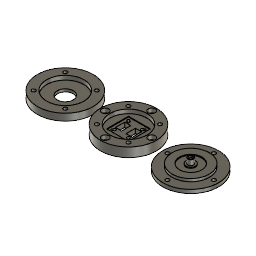
AS5600 holder v2.1 (Autodesk Fusion 360 design; units mm, degrees)
part number: 2026-01-20-22-25-40-409
Autodesk Fusion 360 part; units mm, degrees
sketch "Sketch1" plane through (0, 0, 0) normal (0, 0, 1) x (1, 0, 0)
  circle A0 centre (0, 0) radius 1.9
  circle A1 centre (0, 0) radius 4.9
  circle A2 centre (0, 0) radius 20
  dimension "d1" = 3.8
  dimension "d2" = 9.8
  constraint coincident A0.centre A1.centre
  constraint concentric A0 A1
  constraint concentric A1 A2
  measures "d1" diameter of A0
  measures "d2" diameter of A1
sketch "Sketch2" plane through (0, 0, 0) normal (0, 0, 1) x (1, 0, 0)
  line L0 (30, -30) -> (-30, -30)
  line L1 (-30, -30) -> (-30, 30)
  line L2 (-30, 30) -> (30, 30)
  line L3 (30, 30) -> (30, -30)
  line L4 (30, -30) -> (-30, 30) construction
  line L5 (-30, -30) -> (30, 30) construction
  constraint horizontal L0
  constraint perpendicular L0 L1
  constraint parallel L0 L2
  constraint parallel L1 L3
  constraint coincident L4 origin
  constraint coincident L5 origin
extrude "Extrude1" add sketch "Sketch1" along normal blind 5 contours A0 | A1 | A2 picked at (0.583136, -0.509268) picked at (3.874683, -0.337829) picked at (14.873963, -1.237051) makes body 1
sketch "Sketch3" plane through (0, 0, 0) normal (0, 0, 1) x (1, 0, 0)
extrude "Extrude2" add sketch "Sketch2" along normal blind 3 contours L0 L1 L2 L3 picked at (10, -10) bodies 1
extrude "Extrude3" add sketch "Sketch1" along normal blind 8 contours A0 | A1 picked at (0.583136, -0.509268) picked at (3.874683, -0.337829) bodies 1
sketch "Sketch4" plane through (0, 0, 0) normal (0, 0, 1) x (1, 0, 0)
  circle A0 centre (0, 0) radius 1.9
  dimension "d9" = 3.8
  constraint coincident A0.centre origin
  measures "d9" diameter of A0
sketch "Sketch5" plane through (0, 0, 8) normal (0, 0, 1) x (-1, 0, 0)
  circle A0 centre (0, 0) radius 4.9
  circle A1 centre (0, 0) radius 1.9
  dimension "d10" = 3.8
  constraint coincident A0.centre A1.centre
  measures "d10" diameter of A1
extrude "Extrude4" cut sketch "Sketch5" against normal blind 1 contours A1 picked at (0.583136, -0.509268) bodies 1
sketch "Sketch6" plane through (0, 0, 3) normal (0, 0, 1) x (-1, 0, 0)
  line L0 (-30, -30) -> (30, -30)
  line L1 (30, -30) -> (30, 30)
  line L2 (30, 30) -> (-30, 30)
  line L3 (-30, 30) -> (-30, -30)
  circle A0 centre (0, 0) radius 20
  line L4 (-11.75, -11.75) -> (11.75, -11.75)
  line L5 (11.75, -11.75) -> (11.75, 11.75)
  line L6 (11.75, 11.75) -> (-11.75, 11.75)
  line L7 (-11.75, 11.75) -> (-11.75, -11.75)
  line L8 (-11.75, -11.75) -> (11.75, 11.75) construction
  line L9 (11.75, -11.75) -> (-11.75, 11.75) construction
  line L10 (11.75, -11.75) -> (8.75, -11.75)
  line L11 (8.75, -11.75) -> (8.75, -8.75)
  line L12 (8.75, -8.75) -> (11.75, -8.75)
  line L13 (11.75, -8.75) -> (11.75, -11.75)
  line L14 (-8.75, -11.75) -> (-11.75, -11.75)
  line L15 (-11.75, -11.75) -> (-11.75, -8.75)
  line L16 (-8.75, -8.75) -> (-8.75, -11.75)
  line L17 (-11.75, -8.75) -> (-8.75, -8.75)
  line L18 (11.75, 8.75) -> (8.75, 8.75)
  line L19 (8.75, 8.75) -> (8.75, 11.75)
  line L20 (11.75, 11.75) -> (11.75, 8.75)
  line L21 (8.75, 11.75) -> (11.75, 11.75)
  line L22 (-8.75, 8.75) -> (-11.75, 8.75)
  line L23 (-11.75, 8.75) -> (-11.75, 11.75)
  line L24 (-8.75, 11.75) -> (-8.75, 8.75)
  line L25 (-11.75, 11.75) -> (-8.75, 11.75)
  circle A1 centre (8.75, -8.75) radius 1.06066
  circle A2 centre (-8.75, -8.75) radius 1.06066
  circle A3 centre (8.75, 8.75) radius 1.06066
  circle A4 centre (-8.75, 8.75) radius 1.06066
  dimension "d13" = 23.5
  dimension "d14" = 23.5
  dimension "d15" = 3
  dimension "d16" = 3
  constraint horizontal L4
  constraint perpendicular L4 L5
  constraint parallel L4 L6
  constraint parallel L5 L7
  constraint coincident L8 A0.centre
  constraint coincident L9 A0.centre
  constraint coincident A0.centre origin
  constraint horizontal L10
  constraint vertical L11
  constraint horizontal L12
  constraint vertical L13
  constraint coincident L11.end L12.start
  measures "d13" distance of L4.start L4.end
  measures "d14" distance of L4.start L6.end
  measures "d15" distance of L10.end L11.end
  measures "d16" distance of L11.end L12.end
copy_body "CopyPasteBodies1" bodies 1 makes body 2
move_body "Move1" bodies 2 to x (1, 0, 0) y (0, 1, 0) z (0, 0, 1) at (80, 0, 0)
extrude "Extrude5" add 1 faces at (14.873963, -1.237051, 5) along direction (0, 0, 1) blind 3 on bodies 1 bodies 1
extrude "Extrude6" cut 1 faces at (13.892206, -0.993615, 8) along direction (0, 0, -1) blind 4.8 on bodies 1 bodies 1
extrude "Extrude7" cut 1 faces at (-0.583136, 0.509268, 7) along direction (0, 0, -1) blind 3.85 on bodies 1 bodies 1
extrude "Extrude8" cut sketch "Sketch6" against normal blind 4 contours L16 L17 A2 | L16 L17 A2 | L11 L12 A1 | L11 L12 A1 | L22 L24 A4 | L22 L24 A4 | L18 L19 A3 | L18 L19 A3 picked at (-9.453508, -8.800316) picked at (-8.855094, -8.052746) picked at (8.698123, -9.45328) picked at (9.453508, -8.800316) picked at (-8.899923, 9.439187) picked at (-9.453158, 8.697306) picked at (9.45328, 8.698123) picked at (8.899923, 9.439187) bodies 1
extrude "Extrude9" cut 4 faces at (-8.86162, -8.363997, 3) (8.580058, -9.010844, 3) (8.490827, 9.16775, 3) (-9.256031, 9.066623, 3) along direction (0, 0, 1) blind 4 on bodies 1 bodies 1
extrude "Extrude10" cut 1 faces at (-12.758335, 0, 3.2) along direction (0, 0, -1) blind 0.5 on bodies 1 bodies 1
extrude "Extrude11" cut 1 faces at (-0.583136, 0.509268, 3.15) along direction (0, 0, -1) blind 1 on bodies 1 bodies 1
extrude "Extrude12" cut sketch "Sketch6" against normal blind 1 contours L4 L7 L14 L15 L16 L17 A2 | L4 L5 L6 L7 L11 L12 L16 L17 L18 L19 L22 L24 A1 A2 A3 A4 | L4 L5 L10 L11 L12 L13 A1 | L6 L7 L22 L23 L24 L25 A4 | L5 L6 L18 L19 L20 L21 A3 picked at (-11.047428, -9.941145) picked at (-2.648321, 2.666667) picked at (9.941145, -11.047428) picked at (-11.047428, 9.941145) picked at (9.941145, 11.047428) bodies 1
extrude "Extrude13" cut 1 faces at (83.881757, -0.243436, 8) along direction (0, 0, -1) blind 3 on bodies 2 bodies 2
sketch "Sketch7" plane through (0, 0, 7) normal (0, 0, 1) x (-1, 0, 0)
  circle A0 centre (-80, 0) radius 1.9
  circle A1 centre (-80, 0) radius 3.05
  dimension "d44" = 6.1
  constraint concentric A0 A1
  measures "d44" diameter of A1
extrude "Extrude14" add sketch "Sketch7" against normal blind 2 contours A1 picked at (-80.829042, -2.527118) bodies 2
sketch "Sketch8" plane through (0, 0, 7) normal (0, 0, 1) x (-1, 0, 0)
  circle A0 centre (-80, 0) radius 3.05
  circle A1 centre (-80, 0) radius 1.950002
  constraint concentric A0 A1
extrude "Extrude15" add sketch "Sketch8" along normal blind 5 contours A0 picked at (-80.835132, -2.542633) bodies 2
extrude "Extrude16" cut 1 faces at (80.835132, 2.542633, 12) along direction (0, 0, -1) blind 1 on bodies 2 bodies 2
extrude "Extrude17" cut 1 faces at (80.835132, 2.542633, 11) along direction (0, 0, -1) blind 0.5 on bodies 2 bodies 2
extrude "Extrude18" add 1 faces at (79.41437, 0.282025, 7) along direction (0, 0, 1) blind 2.5 on bodies 2 bodies 2
sketch "Sketch9" plane through (0, 0, 3) normal (0, 0, 1) x (-1, 0, 0)
  line L0 (-30, -30) -> (30, -30)
  line L1 (30, -30) -> (30, 30)
  line L2 (30, 30) -> (-30, 30)
  line L3 (-30, 30) -> (-30, -30)
  circle A0 centre (0, 0) radius 20
  circle A1 centre (0, 0) radius 8.25
  dimension "d55" = 16.5
  constraint concentric A0 A1
  measures "d55" diameter of A1
copy_body "CopyPasteBodies2" bodies 2 makes body 3
move_body "Move2" bodies 3 to x (1, 0, 0) y (0, 1, 0) z (0, 0, 1) at (85, 0, 0)
extrude "Extrude19" cut 1 faces at (162.328021, 0.151526, 10.5) along direction (0, 0, -1) blind 2 on bodies 3 bodies 3
move_face "OffsetFaces1" offset -5 1 faces at (164.41437, 0.282025, 9.5) on bodies 3
move_face "OffsetFaces2" offset -3.5 1 faces at (162.328021, 0.151526, 8.5) on bodies 3
extrude "Extrude20" cut 1 faces at (178.901613, -1.090493, 5) along direction (0, 0, -1) blind 2 on bodies 3 bodies 3
extrude "Extrude21" cut 1 faces at (164.41437, 0.282025, 4.5) along direction (0, 0, -1) blind 1.5 on bodies 3 bodies 3
sketch "Sketch10" plane through (0, 0, 3) normal (0, 0, 1) x (-1, 0, 0)
  line L0 (-195, -30) -> (-135, -30)
  line L1 (-135, -30) -> (-135, 30)
  line L2 (-135, 30) -> (-195, 30)
  line L3 (-195, 30) -> (-195, -30)
  circle A0 centre (-165.000002, 0) radius 8.525
  circle A1 centre (-165.000002, 0) radius 20
  dimension "d67" = 17.05
  constraint concentric A0 A1
  measures "d67" diameter of A0
extrude "Extrude22" cut sketch "Sketch10" against normal blind 7 contours A0 picked at (-163.228252, -3.896896) bodies 3
extrude "Extrude23" add sketch "Sketch10" along normal blind 2 contours A1 picked at (-148.931202, -1.417144) bodies 3
extrude "Extrude24" add 1 faces at (148.931202, 1.417144, 5) along direction (0, 0, 1) blind 1 on bodies 3 bodies 3
sketch "Sketch11" plane through (0, 0, 3) normal (0, 0, 1) x (1, 0, 0)
extrude "Extrude25" cut 1 faces at (148.931202, 1.417144, 6) along direction (0, 0, -1) blind 5 on bodies 3 bodies 3
extrude "Extrude26" add sketch "Sketch10" along normal blind 2 contours L0 L1 L2 L3 picked at (-164.5018, -26.648025) bodies 3
extrude "Extrude27" add sketch "Sketch10" along normal blind 1 contours A1 picked at (-148.931202, -1.417144) bodies 3
move_face "OffsetFaces3" offset -1 1 faces at (148.931202, 1.417144, 4) on bodies 3
extrude "Extrude28" add 1 faces at (148.931202, 1.417144, 1) along direction (0, 0, 1) blind 1 on bodies 3 bodies 3
move_body "Move3" bodies 3 to x (1, 0, 0) y (0, 1, 0) z (0, 0, 1) at (-165, 0, 3)
sketch "Sketch12" plane through (0, 0, 8) normal (0, 0, 1) x (-1, 0, 0)
  circle A0 centre (-0.000002, 0) radius 20
  line L0 (-30, 30) -> (-30, -30)
  line L1 (-30, -30) -> (30, -30)
  line L2 (30, -30) -> (30, 30)
  line L3 (30, 30) -> (-30, 30)
  circle A1 centre (-25, 25) radius 1.5
  circle A2 centre (25, 25) radius 1.5
  circle A3 centre (-25, -25) radius 1.5
  circle A4 centre (25, -25) radius 1.5
  dimension "d88" = 50
  dimension "d89" = -50
extrude "Extrude29" cut sketch "Sketch12" against normal blind 14 contours A1 | A2 | A3 | A4 picked at (-25.41312, 24.986905) picked at (24.58688, 24.986905) picked at (-25.41312, -25.013095) picked at (24.58688, -25.013095) bodies 1 3
sketch "Sketch13" plane through (0, 0, 3) normal (0, 0, 1) x (-1, 0, 0)
  line L0 (-110, -30) -> (-50, -30)
  line L1 (-50, -30) -> (-50, 30)
  line L2 (-50, 30) -> (-110, 30)
  line L3 (-110, 30) -> (-110, -30)
  circle A0 centre (-80, 0) radius 20
  circle A1 centre (-105.000002, 25) radius 1.5
  circle A2 centre (-55.000002, 25) radius 1.5
  circle A3 centre (-105.000002, -25) radius 1.5
  circle A4 centre (-55.000002, -25) radius 1.5
  dimension "d94" = 50
  dimension "d95" = -50
extrude "Extrude30" cut sketch "Sketch13" against normal blind 21 contours A1 | A2 | A3 | A4 picked at (-105.413121, 25.013096) picked at (-55.081298, 24.209935) picked at (-105.413121, -24.986904) picked at (-55.081298, -25.790065) bodies 2
move_body "Move4" bodies 2 to x (0, -1, 0) y (1, 0, 0) z (0, 0, 1) at (80, 80, 0)
move_body "Move5" bodies 2 to x (1, 0, 0) y (0, 1, 0) z (0, 0, 1) at (-80, 0, 13)
move_body "Move6" bodies 2 to x (1, 0, 0) y (0, -1, 0) z (0, 0, -1) at (0, -60, 16)
move_body "Move7" bodies 2 to x (1, 0, 0) y (0, 1, 0) z (0, 0, 1) at (0, 60, 8)
move_body "Move8" bodies 2 to x (1, 0, 0) y (0, 1, 0) z (0, 0, 1) at (0, 0, 3)
move_body "Move9" bodies 2 to x (1, 0, 0) y (0, 1, 0) z (0, 0, 1) at (0, 0, 1)
extrude "Extrude31" add 1 faces at (0.498201, -24.180718, 3) along direction (0, 0, 1) blind 1 on bodies 1 bodies 1
extrude "Extrude32" add 1 faces at (-16.068798, 1.417144, 5) along direction (0, 0, 1) blind 1 on bodies 3 bodies 3
move_body "Move10" bodies 1 to x (1, 0, 0) y (0, 1, 0) z (0, 0, 1) at (0, 0, -1)
move_face "MoveFace1" by (0, 0, -1) 1 faces at (-0.993615, 14.275539, 10) on bodies 2
move_body "Move11" bodies 2 to x (1, 0, 0) y (0, 1, 0) z (0, 0, 1) at (0, 0, 3)
move_face "OffsetFaces4" offset 1 1 faces at (-24.180718, 0.498202, 15) on bodies 2
move_body "Move12" bodies 2 to x (1, 0, 0) y (0, 1, 0) z (0, 0, 1) at (0, 0, -5)
move_body "Move13" bodies 1 to x (1, 0, 0) y (0, 1, 0) z (0, 0, 1) at (0, 0, -1)
move_face "OffsetFaces5" offset 1 1 faces at (20.284924, -2.807413, -2) on bodies 1
extrude "Extrude33" cut 1 faces at (2.657494, 2.676189, 0) along direction (0, 0, -1) blind 1 on bodies 1 bodies 1
move_body "Move14" bodies 1 to x (1, 0, 0) y (0, 1, 0) z (0, 0, 1) at (65, 0, 0)
move_body "Move15" bodies 2 to x (1, 0, 0) y (0, 1, 0) z (0, 0, 1) at (-70, 0, 0)
move_body "Move16" bodies 2 to x (-1, 0, 0) y (0, 1, 0) z (0, 0, -1) at (-200, 0, 26)
move_body "Move17" bodies 3 to x (1, 0, 0) y (0, 1, 0) z (0, 0, 1) at (0, 0, -6)
move_body "Move18" bodies 2 to x (1, 0, 0) y (0, 1, 0) z (0, 0, 1) at (60, 0, -16)
move_body "Move19" bodies 2 to x (1, 0, 0) y (0, 1, 0) z (0, 0, 1) at (5, 0, 0)
sketch "Sketch14" plane through (0, 0, 6.5) normal (0, 0, 1) x (-1, 0, 0)
  circle A0 centre (65, 0) radius 1.950002
  circle A1 centre (65, 0) radius 2.1
  dimension "d151" = 4.2
  constraint concentric A0 A1
  measures "d151" diameter of A1
extrude "Extrude34" cut sketch "Sketch14" along normal blind 2.8 contours A1 picked at (63.017795, 0.502249) bodies 2
fillet "Fillet1" radius 0.2 1 edges at (-63.042113, -0.759392, 7.5) on bodies 2
move_face "OffsetFaces6" offset -0.5 1 faces at (-65.57464, -0.884169, 6.5) on bodies 2
sketch "Sketch15" plane through (0, 0, 7.5) normal (0, 0, 1) x (-1, 0, 0)
  circle A0 centre (65, 0) radius 3.05
  circle A1 centre (65, 0) radius 2.3
  circle A2 centre (65, 0) radius 3.150001
  constraint concentric A0 A2
move_body "Move20" bodies 2 to x (1, 0, 0) y (0, 1, 0) z (0, 0, 1) at (0, 0, 5)
extrude "Extrude35" add sketch "Sketch15" along normal blind 3 contours A0 | A1 | A2 picked at (64.122246, 2.651235) picked at (65.383333, 0.663953) picked at (62.079131, -1.064739) bodies 2
sketch "Sketch16" plane through (0, 0, 8) normal (0, 0, 1) x (-1, 0, 0)
  circle A0 centre (65, 0) radius 3.150001
  circle A1 centre (65, 0) radius 20
  circle A2 centre (65, 0) radius 5.05
  circle A3 centre (65, 0) radius 11.999999
  dimension "d162" = 10.1
  constraint concentric A0 A2
  constraint concentric A2 A3
  measures "d162" diameter of A2
extrude "Extrude36" cut sketch "Sketch16" against normal blind 1 contours A3 picked at (74.619855, -0.847057) bodies 2
move_body "Move21" bodies 2 to x (1, 0, 0) y (0, 1, 0) z (0, 0, 1) at (0, 0, -5)
sketch "Sketch17" plane through (0, 0, -1) normal (0, 0, 1) x (-1, 0, 0)
  circle A0 centre (-56.25, 8.75) radius 1.06066
  circle A1 centre (-56.25, -8.75) radius 1.06066
  circle A2 centre (-73.75, 8.75) radius 1.06066
  circle A3 centre (-73.75, -8.75) radius 1.06066
  line L0 (-76.75, 11.75) -> (-76.75, -11.75)
  line L1 (-76.75, -11.75) -> (-53.25, -11.75)
  line L2 (-53.25, -11.75) -> (-53.25, 11.75)
  line L3 (-53.25, 11.75) -> (-76.75, 11.75)
  circle A4 centre (-57.500001, 7.5) radius 1.5
  circle A5 centre (-72.500001, 7.5) radius 1.5
  circle A6 centre (-57.500001, -7.5) radius 1.5
  circle A7 centre (-72.500001, -7.5) radius 1.5
  dimension "d170" = -15
  dimension "d171" = -15
extrude "Extrude37" cut sketch "Sketch17" against normal blind 8 contours A0 A4 | A1 A6 | A2 A5 | A3 A7 picked at (-58.0875, 7.014111) picked at (-58.0875, -7.014111) picked at (-71.97808, 6.946261) picked at (-71.97808, -6.946261) bodies 1
move_body "Move22" bodies 3 to x (1, 0, 0) y (0, 1, 0) z (0, 0, 1) at (65, 0, 10)
move_body "Move23" bodies 2 to x (1, 0, 0) y (0, 1, 0) z (0, 0, 1) at (130, 0, 20)
sketch "Sketch18" plane through (0, 0, 0) normal (0, 0, 1) x (1, 0, 0)
  circle A0 centre (65, 0) radius 40
  circle A1 centre (65, 0) radius 45
  constraint concentric A0 A1
extrude "Extrude38" cut sketch "Sketch18" along normal mid plane 90 contours A0 picked at (74.48469, -14.222306) keep common part bodies 1 2 3
move_body "Move24" bodies 2 to x (1, 0, 0) y (0, 1, 0) z (0, 0, 1) at (65, 0, -20)
move_body "Move25" bodies 3 to x (1, 0, 0) y (0, 1, 0) z (0, 0, 1) at (-65, 0, -10)
move_face "OffsetFaces7" offset -0.1 1 faces at (129.921468, -3.149022, 3.833333) on bodies 2
extrude "Extrude39" add 1 faces at (130.578367, -0.394324, 6) along direction (0, 0, 1) blind 2 on bodies 2 bodies 2
extrude "Extrude40" add 1 faces at (130.335716, -2.764868, 7.5) along direction (0, 0, 1) blind 2 on bodies 2 bodies 2
move_face "OffsetFaces8" offset 5 1 faces at (85.274348, -2.779056, -3) on bodies 1
sketch "Sketch19" plane through (0, 0, 2) normal (0, 0, 1) x (-1, 0, 0)
  circle A0 centre (-65, 0) radius 20
  arc A1 (-38.542487, -30) -> (-35, -26.457513) centre (-65, 0) ccw
  line L0 (-35, -26.457513) -> (-35, 26.457513)
  arc A2 (-35, 26.457513) -> (-38.542487, 30) centre (-65, 0) ccw
  line L1 (-38.542487, 30) -> (-91.457513, 30)
  arc A3 (-91.457513, 30) -> (-95, 26.457513) centre (-65, 0) ccw
  line L2 (-95, 26.457513) -> (-95, -26.457513)
  arc A4 (-95, -26.457513) -> (-91.457513, -30) centre (-65, 0) ccw
  line L3 (-91.457513, -30) -> (-38.542487, -30)
  circle A5 centre (-90, -25) radius 1.5
  circle A6 centre (-90, 25) radius 1.5
  circle A7 centre (-40, -25) radius 1.5
  circle A8 centre (-40, 25) radius 1.5
  circle A9 centre (-65.000001, 25) radius 2
  circle A10 centre (-90, -0.000001) radius 2
  circle A11 centre (-64.999999, -25) radius 2
  circle A12 centre (-40, 0.000001) radius 2
  dimension "d195" = 360
extrude "Extrude41" cut sketch "Sketch19" against normal blind 44 contours A9 | A10 | A11 | A12 picked at (-65.63705, 24.803497) picked at (-89.95018, -1.05781) picked at (-65.637048, -25.196504) picked at (-39.58434, -0.385675) bodies 1
move_body "Move26" bodies 1 to x (1, 0, 0) y (0, 1, 0) z (0, 0, 1) at (0, 0, 5)
sketch "Sketch20" plane through (0, 0, 4) normal (0, 0, 1) x (-1, 0, 0)
  arc A0 (-56.015572, -7.715571) -> (-57.284429, -8.984428) centre (-57.500001, -7.5) ccw
  arc A1 (-57.284429, -8.984428) -> (-56.015572, -7.715571) centre (-56.25, -8.75) ccw
  arc A2 (-57.284429, 8.984429) -> (-56.015572, 7.715571) centre (-57.500001, 7.5) ccw
  arc A3 (-56.015572, 7.715571) -> (-57.284429, 8.984429) centre (-56.25, 8.75) ccw
  arc A4 (-73.984429, 7.715571) -> (-72.715571, 8.984429) centre (-72.500001, 7.5) ccw
  arc A5 (-72.715571, 8.984429) -> (-73.984429, 7.715571) centre (-73.75, 8.75) ccw
  arc A6 (-72.715571, -8.984429) -> (-73.984429, -7.715571) centre (-72.500001, -7.5) ccw
  arc A7 (-73.984429, -7.715571) -> (-72.715571, -8.984429) centre (-73.75, -8.75) ccw
  line L0 (-76.75, 11.75) -> (-76.75, -11.75)
  line L1 (-76.75, -11.75) -> (-53.25, -11.75)
  line L2 (-53.25, -11.75) -> (-53.25, 11.75)
  line L3 (-53.25, 11.75) -> (-76.75, 11.75)
  line L4 (-56.000001, -5) -> (-60.000001, -5)
  line L5 (-60.000001, -5) -> (-60.000001, 5)
  line L6 (-60.000001, 5) -> (-56.000001, 5)
  line L7 (-56.000001, 5) -> (-56.000001, -5)
  line L8 (-70.000001, -5) -> (-74.000001, -5)
  line L9 (-74.000001, -5) -> (-74.000001, 5)
  line L10 (-74.000001, 5) -> (-70.000001, 5)
  line L11 (-70.000001, 5) -> (-70.000001, -5)
  constraint horizontal L4
  constraint vertical L5
  constraint horizontal L6
  constraint vertical L7
  constraint horizontal L8
  constraint vertical L9
  constraint horizontal L10
  constraint vertical L11
extrude "Extrude42" cut sketch "Sketch20" against normal blind 8 contours L4 L5 L6 L7 | L8 L9 L10 L11 picked at (-57.333334, -1.666667) picked at (-71.333334, -1.666667) bodies 1
extrude "Extrude43" cut 1 faces at (66.666668, -1.666667, 4) along direction (0, 0, -1) blind 2 on bodies 1 bodies 1
extrude "Extrude44" cut 1 faces at (50.5, 0, 5.7) along direction (0, 0, -1) blind 3 on bodies 1 bodies 1
sketch "Sketch21" plane through (0, 0, 2) normal (0, 0, 1) x (-1, 0, 0)
  line L0 (-60.000001, -5) -> (-60.000001, 5)
  line L1 (-60.000001, 5) -> (-56.000001, 5)
  line L2 (-56.000001, 5) -> (-56.000001, -5)
  line L3 (-56.000001, -5) -> (-60.000001, -5)
  line L4 (-74.000001, -5) -> (-74.000001, 5)
  line L5 (-74.000001, 5) -> (-70.000001, 5)
  line L6 (-70.000001, 5) -> (-70.000001, -5)
  line L7 (-70.000001, -5) -> (-74.000001, -5)
  arc A0 (-56.015572, -7.715571) -> (-57.284429, -8.984428) centre (-57.500001, -7.5) ccw
  arc A1 (-57.284429, -8.984428) -> (-56.015572, -7.715571) centre (-56.25, -8.75) ccw
  arc A2 (-57.284429, 8.984429) -> (-56.015572, 7.715571) centre (-57.500001, 7.5) ccw
  arc A3 (-56.015572, 7.715571) -> (-57.284429, 8.984429) centre (-56.25, 8.75) ccw
  arc A4 (-73.984429, 7.715571) -> (-72.715571, 8.984429) centre (-72.500001, 7.5) ccw
  arc A5 (-72.715571, 8.984429) -> (-73.984429, 7.715571) centre (-73.75, 8.75) ccw
  arc A6 (-72.715571, -8.984429) -> (-73.984429, -7.715571) centre (-72.500001, -7.5) ccw
  arc A7 (-73.984429, -7.715571) -> (-72.715571, -8.984429) centre (-73.75, -8.75) ccw
  line L8 (-76.75, 11.75) -> (-76.75, -11.75)
  line L9 (-76.75, -11.75) -> (-53.25, -11.75)
  line L10 (-53.25, -11.75) -> (-53.25, 11.75)
  line L11 (-53.25, 11.75) -> (-76.75, 11.75)
  line L12 (-60.000001, -5) -> (-62.500001, -5)
  line L13 (-62.500001, -5) -> (-62.500001, 5)
  line L14 (-62.500001, 5) -> (-60.000001, 5)
  line L15 (-60.000001, 5) -> (-60.000001, -5)
  line L16 (-70.000001, -5) -> (-67.500001, -5)
  line L17 (-67.500001, -5) -> (-67.500001, 5)
  line L18 (-67.500001, 5) -> (-70.000001, 5)
  line L19 (-70.000001, 5) -> (-70.000001, -5)
  constraint horizontal L12
  constraint vertical L13
  constraint horizontal L14
  constraint vertical L15
  constraint horizontal L16
  constraint vertical L17
  constraint horizontal L18
  constraint vertical L19
extrude "Extrude45" cut sketch "Sketch21" against normal blind 11.5 contours L0 L12 L13 L14 L15 | L6 L16 L17 L18 L19 picked at (-60.833334, -1.666667) picked at (-69.166668, 1.666667) bodies 1
move_body "Move27" bodies 2 to x (1, 0, 0) y (0, 1, 0) z (0, 0, 1) at (-65, 15, 10)
move_body "Move28" bodies 2 to x (1, 0, 0) y (0, 1, 0) z (0, 0, 1) at (0, -15, 0)
sketch "Sketch22" plane through (0, 0, 11) normal (0, 0, 1) x (-1, 0, 0)
  circle A0 centre (-65, 0) radius 20
  arc A1 (-38.542487, -30) -> (-35, -26.457513) centre (-65, 0) ccw
  line L0 (-35, -26.457513) -> (-35, 26.457513)
  arc A2 (-35, 26.457513) -> (-38.542487, 30) centre (-65, 0) ccw
  line L1 (-38.542487, 30) -> (-91.457513, 30)
  arc A3 (-91.457513, 30) -> (-95, 26.457513) centre (-65, 0) ccw
  line L2 (-95, 26.457513) -> (-95, -26.457513)
  arc A4 (-95, -26.457513) -> (-91.457513, -30) centre (-65, 0) ccw
  line L3 (-91.457513, -30) -> (-38.542487, -30)
  circle A5 centre (-40, 24.999998) radius 1.5
  circle A6 centre (-40, -25.000002) radius 1.5
  circle A7 centre (-90, 24.999998) radius 1.5
  circle A8 centre (-90, -25.000002) radius 1.5
  circle A9 centre (-40.000001, 0) radius 2
  circle A10 centre (-65, 24.999999) radius 2
  circle A11 centre (-89.999999, 0) radius 2
  circle A12 centre (-65, -24.999999) radius 2
  dimension "d216" = 360
extrude "Extrude46" cut sketch "Sketch22" against normal blind 8 contours A9 | A10 | A11 | A12 picked at (-39.584341, -0.385676) picked at (-65.637049, 24.803496) picked at (-89.950179, -1.057809) picked at (-65.637049, -25.196503) bodies 2
move_body "Move29" bodies 2 to x (1, 0, 0) y (0, 1, 0) z (0, 0, 1) at (70, 0, -10)
move_body "Move30" bodies 3 to x (1, 0, 0) y (0, 1, 0) z (0, 0, 1) at (-4, 0, 0)
move_body "Move31" bodies 1 to x (1, 0, 0) y (0, 0, 1) z (0, -1, 0) at (0, -23, 37)
move_body "Move32" bodies 1 to x (1, 0, 0) y (0, 0, -1) z (0, 1, 0) at (0, -27, -13)
move_body "Move33" bodies 1 to x (1, 0, 0) y (0, 1, 0) z (0, 0, 1) at (0, 0, -10)
move_body "Move34" bodies 1 to x (1, 0, 0) y (0, 1, 0) z (0, 0, 1) at (0, -10, 0)
extrude "Extrude47" add 1 faces at (-4.4982, 26.648025, 2) along direction (0, 0, 1) blind 2.5 on bodies 3 bodies 3
move_body "Move35" bodies 1 to x (1, 0, 0) y (0, 1, 0) z (0, 0, 1) at (-69, 0, 0)
move_body "Move36" bodies 1 to x (1, 0, 0) y (0, 1, 0) z (0, 0, 1) at (0, 5, 10)
move_body "Move37" bodies 2 to x (1, 0, 0) y (0, 1, 0) z (0, 0, 1) at (-138, 0, 30)
move_body "Move38" bodies 1 to x (1, 0, 0) y (0, 1, 0) z (0, 0, 1) at (63, -5, 0)
move_body "Move39" bodies 2 to x (1, 0, 0) y (0, 1, 0) z (0, 0, 1) at (-1, 0, 0)
move_body "Move40" bodies 1 to x (1, 0, 0) y (0, 1, 0) z (0, 0, 1) at (-63, 0, 0)
move_body "Move41" bodies 1 to x (1, 0, 0) y (0, 1, 0) z (0, 0, 1) at (0, 0, 2)
sketch "Sketch23" plane through (0, 0, 31) normal (0, 0, 1) x (-1, 0, 0)
  circle A0 centre (4, -24.999999) radius 2
  circle A1 centre (-20.999999, 0) radius 2
  circle A2 centre (28.999999, 0) radius 2
  circle A3 centre (4, 24.999999) radius 2
  circle A4 centre (4, 0) radius 20
  arc A5 (30.457513, -30) -> (34, -26.457513) centre (4, 0) ccw
  line L0 (34, -26.457513) -> (34, 26.457513)
  arc A6 (34, 26.457513) -> (30.457513, 30) centre (4, 0) ccw
  line L1 (30.457513, 30) -> (-22.457513, 30)
  arc A7 (-22.457513, 30) -> (-26, 26.457513) centre (4, 0) ccw
  line L2 (-26, 26.457513) -> (-26, -26.457513)
  arc A8 (-26, -26.457513) -> (-22.457513, -30) centre (4, 0) ccw
  line L3 (-22.457513, -30) -> (30.457513, -30)
  circle A9 centre (29, 24.999998) radius 1.5
  circle A10 centre (29, -25.000002) radius 1.5
  circle A11 centre (-21, 24.999998) radius 1.5
  circle A12 centre (-21, -25.000002) radius 1.5
  circle A13 centre (4, 0) radius 30
  constraint concentric A4 A13
  constraint tangent L2 A13
extrude "Extrude48" cut sketch "Sketch23" against normal blind 47 contours A5 L0 L3 A13 | L2 A8 L3 A13 | L0 A6 L1 A13 | L1 A7 L2 A13 picked at (31.508855, -18.379729) picked at (-23.508855, -18.379729) picked at (22.379729, 27.508855) picked at (-23.508855, 18.379729) bodies 1 2 3
move_body "Move42" bodies 2 to x (1, 0, 0) y (0, 1, 0) z (0, 0, 1) at (135, 0, -30)
move_face "OffsetFaces9" offset 0.1 1 faces at (131.399391, 2.265058, 8.833333) on bodies 2
sketch "Sketch24" plane through (0, 0, 19) normal (0, 0, 1) x (-1, 0, 0)
  circle A0 centre (4, 0) radius 30
  circle A1 centre (29, 0.000001) radius 2
  circle A2 centre (4.000001, -25) radius 2
  circle A3 centre (3.999999, 25) radius 2
  circle A4 centre (-21, -0.000001) radius 2
  circle A5 centre (4, 0) radius 20
  circle A6 centre (3.999999, 25) radius 1.999999
  circle A7 centre (-21, -0.000001) radius 1.999999
  circle A8 centre (4.000001, -25) radius 1.999999
  circle A9 centre (29, 0.000001) radius 1.999999
  dimension "d263" = 360
  constraint concentric A3 A6
sketch "Sketch25" plane through (0, 0, 19) normal (0, 0, 1) x (-1, 0, 0)
  line L0 (-8, -12) -> (16, -12)
  line L1 (16, -12) -> (16, 12)
  line L2 (16, 12) -> (-8, 12)
  line L3 (-8, 12) -> (-8, -12)
  line L4 (-8, -12) -> (16, 12) construction
  line L5 (16, -12) -> (-8, 12) construction
  point P0 (4, 0)
  constraint horizontal L0
  constraint perpendicular L0 L1
  constraint parallel L0 L2
  constraint parallel L1 L3
  constraint coincident L4 P0
  constraint coincident L5 P0
sketch "Sketch26" plane through (0, 0, 19) normal (0, 0, 1) x (-1, 0, 0)
sketch "Sketch27" plane through (0, 0, 19) normal (0, 0, 1) x (-1, 0, 0)
  line L0 (29, 0) -> (4, 0)
  line L1 (4, 0) -> (4, 25)
  line L2 (4, 25) -> (29, 25)
  line L3 (29, 25) -> (29, 0)
  line L4 (29, 25) -> (21, 25)
  line L5 (21, 25) -> (21, 17)
  line L6 (21, 17) -> (29, 17)
  line L7 (29, 17) -> (29, 25)
  circle A0 centre (21, 17) radius 2
  circle A1 centre (-13, 17) radius 2
  circle A2 centre (-13, -17) radius 2
  circle A3 centre (21, -17) radius 2
  dimension "d265" = 360
  constraint horizontal L0
  constraint vertical L1
  constraint horizontal L2
  constraint vertical L3
  constraint horizontal L4
  constraint vertical L5
  constraint horizontal L6
  constraint vertical L7
  constraint coincident L5.end L6.start
extrude "Extrude49" cut sketch "Sketch27" against normal blind 41 contours L5 L6 A0 | L5 L6 A0 | A1 | A2 | A3 picked at (22.326118, 16.90218) picked at (21.282699, 18.299543) picked at (-13.066021, 17.44862) picked at (-12.851653, -17.591213) picked at (21.148348, -17.591213) bodies 1 3
move_body "Move43" bodies 1 to x (1, 0, 0) y (0, 1, 0) z (0, 0, 1) at (68, 0, -12)
move_face "OffsetFaces10" offset 1 1 faces at (129.707465, 17.247687, 3) on bodies 2
move_face "OffsetFaces11" offset 1 1 faces at (132.964991, -3.90524, 3) on bodies 2
move_face "OffsetFaces12" offset 1 1 faces at (121.380145, 0.847057, 2) on bodies 2
sketch "Sketch28" plane through (0, 0, 7) normal (0, 0, 1) x (-1, 0, 0)
  circle A0 centre (-81, 17) radius 2
  circle A1 centre (-81, -17) radius 2
  circle A2 centre (-47, 17) radius 2
  circle A3 centre (-47, -17) radius 2
  circle A4 centre (-64, 0) radius 30
  circle A5 centre (-39, 0.000001) radius 2
  circle A6 centre (-63.999999, -25) radius 2
  circle A7 centre (-64.000001, 25) radius 2
  circle A8 centre (-89, -0.000001) radius 2
  circle A9 centre (-64, 0) radius 20
  circle A10 centre (-63.999999, -25) radius 3.7
  circle A11 centre (-39, 0.000001) radius 3.7
  circle A12 centre (-64.000001, 25) radius 3.7
  circle A13 centre (-89, -0.000001) radius 3.7
  dimension "d274" = 7.4
  dimension "d276" = 360
  constraint concentric A6 A10
  measures "d274" diameter of A10
extrude "Extrude50" cut sketch "Sketch28" against normal blind 4 contours A10 | A11 | A12 | A13 picked at (-66.161768, -27.256587) picked at (-35.880442, -0.183818) picked at (-60.880443, 24.816182) picked at (-90.801298, 2.553577) bodies 1
move_face "OffsetFaces13" offset -0.5 4 faces at (60.880443, -24.816182, 3) (90.801298, -2.553577, 3) (66.161768, 27.256587, 3) (35.880442, 0.183818, 3) on bodies 1
move_body "Move44" bodies 1 to x (-1, 0, 0) y (0, 1, 0) z (0, 0, -1) at (124, 0, 3)
sketch "Sketch29" plane through (0, 0, 6) normal (0, 0, 1) x (-1, 0, 0)
  circle A0 centre (-43, 17) radius 2
  circle A1 centre (-43, -17) radius 2
  circle A2 centre (-77, 17) radius 2
  circle A3 centre (-77, -17) radius 2
  circle A4 centre (-60, 0) radius 30
  line L0 (-62.499999, -5) -> (-68.999999, -5)
  line L1 (-68.999999, -5) -> (-68.999999, 5)
  line L2 (-68.999999, 5) -> (-62.499999, 5)
  line L3 (-62.499999, 5) -> (-62.499999, -5)
  line L4 (-57.499999, 5) -> (-50.999999, 5)
  line L5 (-50.999999, 5) -> (-50.999999, -5)
  line L6 (-50.999999, -5) -> (-57.499999, -5)
  line L7 (-57.499999, -5) -> (-57.499999, 5)
  circle A5 centre (-85, 0.000001) radius 2
  circle A6 centre (-60.000001, -25) radius 2
  circle A7 centre (-59.999999, 25) radius 2
  circle A8 centre (-35, -0.000001) radius 2
  arc A9 (-52.284429, 8.984429) -> (-51.015571, 7.715571) centre (-52.499999, 7.5) ccw
  arc A10 (-51.015571, 7.715571) -> (-52.284429, 8.984429) centre (-51.25, 8.75) ccw
  arc A11 (-51.015571, -7.715571) -> (-52.284429, -8.984429) centre (-52.499999, -7.5) ccw
  arc A12 (-52.284429, -8.984429) -> (-51.015571, -7.715571) centre (-51.25, -8.75) ccw
  arc A13 (-68.984428, 7.715571) -> (-67.715571, 8.984429) centre (-67.499999, 7.5) ccw
  arc A14 (-67.715571, 8.984429) -> (-68.984428, 7.715571) centre (-68.75, 8.75) ccw
  arc A15 (-67.715571, -8.984428) -> (-68.984428, -7.715571) centre (-67.499999, -7.5) ccw
  arc A16 (-68.984428, -7.715571) -> (-67.715571, -8.984428) centre (-68.75, -8.75) ccw
  circle A17 centre (-43, 17) radius 3.7
  circle A18 centre (-77, 17) radius 3.7
  circle A19 centre (-77, -17) radius 3.7
  circle A20 centre (-43, -17) radius 3.7
  dimension "d280" = 7.4
  dimension "d282" = 360
  constraint concentric A0 A17
  measures "d280" diameter of A17
extrude "Extrude51" cut sketch "Sketch29" against normal blind 4.5 contours A17 | A18 | A19 | A20 picked at (-39.887888, 16.71682) picked at (-74.10962, 15.81209) picked at (-74.073217, -18.095158) picked at (-40.109619, -15.81209) bodies 1
move_body "Move45" bodies 1 to x (-1, 0, 0) y (0, 1, 0) z (0, 0, -1) at (120, 0, 6)
move_body "Move46" bodies 3 to x (1, 0, 0) y (0, 1, 0) z (0, 0, 1) at (0, 0, 3)
move_body "Move47" bodies 2 to x (1, 0, 0) y (0, 1, 0) z (0, 0, 1) at (0, 0, 3)
move_body "Move48" bodies 1 to x (1, 0, 0) y (0, 1, 0) z (0, 0, 1) at (4, 0, 0)
move_face "OffsetFaces14" offset 0.1 1 faces at (132.003663, -1.957718, 11.148803) on bodies 2
named bodies: "AS6500", "Magnet holder", "needle bearing holder"
